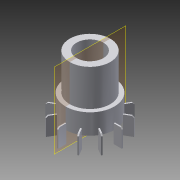
# Autodesk Inventor part: Cooling fan
Saved by Autodesk Inventor 2015 (Build 190141000, 141)
## iProperties
Created: 2008-06-15
Part Number: Cooling fan
Document SubType Name: Modeling
Designer: tangg
Density: 1.4 g/cm^3
Mass: 5.22571 g
Surface Area: 24.131 cm^2
Volume: 5.22571 cm^3
Stock Number: Cooling fan
Material: PVC-U
Appearance: Snow
Author: tangg
Autodesk Inventor part; units mm, degrees
ref_plane "XZ Plane" through (0, 0, 0) normal (0, 1, 0) x (-1, 0, 0)
ref_plane "XY Plane" through (0, 0, 0) normal (0, 0, 1) x (1, 0, 0)
sketch "Sketch1" plane through (0, 0, 0) normal (0, 0, 1) x (1, 0, 0)
  line L0 (0, 0) -> (7.9375, 0)
  line L1 (7.9375, 0) -> (7.9375, -14.2875)
  line L2 (7.9375, -14.2875) -> (0, -14.2875)
  line L3 (0, -14.2875) -> (0, 0)
  line L4 (0, -14.2875) -> (9.525, -14.2875)
  line L5 (9.525, -14.2875) -> (9.525, -22.225)
  line L6 (9.525, -22.225) -> (0, -22.225)
  line L7 (0, -22.225) -> (0, -14.2875)
  constraints: 16 end point
revolve "Revolution1" add sketch "Sketch1" angle 360 about axis through (0, -14.2875, 0) along (0, 1, 0)
sketch "Sketch2" plane through (0, 0, 0) normal (1, 0, 0) x (0, 1, 0)
  line L0 (-14.2875, 7.9375) -> (-14.2875, -7.9375) projected
  line L1 (0, 7.9375) -> (0, -7.9375) projected
  line L2 (-14.2875, -9.525) -> (-22.225, -9.525) projected
  line L3 (-19.8307, -9.525) -> (-26.8886, -9.525)
  line L4 (-26.8886, -9.525) -> (-26.8886, -12.7)
  line L5 (-26.8886, -12.7) -> (-20.4657, -12.7)
  line L6 (-19.8307, -12.065) -> (-19.8307, -9.525)
  line L7 (-20.4657, -12.7) -> (-19.8307, -12.065)
  point P0 (0, 0)
  point P1 (-19.8307, -12.7)
  dimension "d1" = 0.635
  dimension "d2" = 0.635
  constraints: 10 end point, 3 point on line
  measures "d1" distance of L5.end point (-19.831, -12.7)
  measures "d2" distance of L6.start point (-19.831, -12.7)
extrude "Extrusion1" add sketch "Sketch2" along normal mid plane 0.508
pattern_circular "Circular Pattern1" count 12 over 360 about axis through (0, -18.2563, 0) along (0, -1, 0) of "Extrusion1"
sketch "Sketch3" plane through (0, 0, 0) normal (0, 1, 0) x (1, 0, 0)
  circle A0 centre (0, 0) radius 5.25
  dimension "d10" = 10.5
  constraints: 1 centre point, 1 coincident
  measures "d10" diameter of A0
extrude "Extrusion2" cut sketch "Sketch3" against normal through all
equation "\"d2\" = d1"
body "Solid1"
